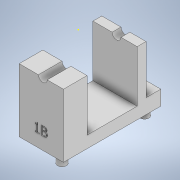
# Autodesk Inventor part: Support_1B
Saved by Autodesk Inventor 2021 (Build 250183000, 183)
## iProperties
Created: 2021-04-14
Part Number: Support_1B
Material: Generic
Document SubType Name: Modeling
Designer: Jawal
Density: 1 g/cm^3
Appearance: Default
Author: Jawal
Autodesk Inventor part; units mm, degrees
note: some values were not read from the file. Chosen so that the rebuilt part matches the saved one: direction of "Emboss1".
ref_plane "YZ Plane" through (0, 0, 0) normal (1, 0, 0) x (0, 1, 0)
ref_plane "XZ Plane" through (0, 0, 0) normal (0, 1, 0) x (-1, 0, 0)
ref_plane "XY Plane" through (0, 0, 0) normal (0, 0, 1) x (1, 0, 0)
sketch "Sketch1" plane through (0, 0, 0) normal (1, 0, 0) x (0, 1, 0)
  line L0 (12.0091, 20) -> (-9.4679, 20)
  line L1 (-9.4679, 20) -> (-9.4679, -13)
  line L2 (-9.4679, -13) -> (12.0091, -13)
  line L3 (12.0091, -13) -> (12.0091, 20)
  point P0 (0, 0)
  dimension "d0" = 33
  dimension "d1" = 21.477
  dimension "d14" = 20
  constraints: 8 end point, 2 parallel, 1 horizontal, 1 perpendicular
  measures "d0" distance of L0.end L1.end
  measures "d1" distance of L1.end L2.end
  measures "d14" distance from line of L0 point (0, 0)
extrude "Extrusion1" add sketch "Sketch1" along normal blind 15
sketch "Sketch2" plane through (0, -9.4679, -13) normal (0, -1, 0) x (1, 0, 0)
  circle A0 centre (12, 30.5) radius 1.5
  line L0 (0, 33) -> (15, 33) projected
  circle A1 centre (12, 2.5) radius 1.5
  line L1 (15, 33) -> (15, 0) projected
  point P0 (0, 13)
  dimension "d4" = 3
  dimension "d5" = 2.5
  dimension "d6" = 3
  dimension "d7" = 28
  dimension "d8" = 3
  dimension "d9" = 3
  constraints: 2 centre point
  measures "d4" diameter of A0
  measures "d5" distance from line of L0 A0.centre
  measures "d6" diameter of A1
  measures "d7" distance of A0.centre A1.centre
  measures "d8" distance from line of A1.centre L1
  measures "d9" distance from line of L1 A0.centre
extrude "Extrusion2" add sketch "Sketch2" along normal blind 3
sketch "Sketch3" plane through (15, 0, 0) normal (1, 0, 0) x (0, 0, -1)
  line L0 (13, 12.0091) -> (-20, 12.0091) projected
  line L1 (-12, 12.0091) -> (5, 12.0091)
  line L2 (5, 12.0091) -> (5, -5.48)
  line L3 (5, -5.48) -> (-12, -5.48)
  line L4 (-12, -5.48) -> (-12, 12.0091)
  line L5 (-20, 12.0091) -> (-20, -9.4679) projected
  line L6 (13, -9.4679) -> (13, 12.0091) projected
  point P0 (0, 0)
  point P1 (5, 12.0091)
  dimension "d12" = 8
  dimension "d13" = 8
  constraints: 8 end point, 2 parallel, 1 horizontal, 1 perpendicular, 1 point on line
  measures "d12" distance between parallel lines of L5 L4
  measures "d13" distance between parallel lines of L6 L2
extrude "Extrusion3" cut sketch "Sketch3" against normal through all
sketch "Sketch4" plane through (0, -9.4679, -13) normal (0, 0, -1) x (-1, 0, 0)
  line L0 (0, 21.477) -> (-15, 21.477) projected
  arc A0 (-9.517, 21.477) -> (-6.517, 21.477) centre (-8.017, 21.477) ccw
  line L1 (-15, 0) -> (-15, 21.477) projected
  point P0 (0, 9.4679)
  dimension "d17" = 3
  dimension "d18" = 6.983
  constraints: 3 point on line, 2 point on circle, 1 centre point
  measures "d17" diameter of A0
  measures "d18" distance from line of L1 A0.centre
extrude "Extrusion4" cut sketch "Sketch4" against normal through all
sketch "Sketch5" plane through (0, 12.0091, -5) normal (0, 1, 0) x (1, 0, 0)
  point P0 (0, -5)
sketch "Sketch6" plane through (0, -9.4679, -13) normal (0, 0, -1) x (-1, 0, 0)
  line L0 (-9.517, 21.477) -> (-15, 21.477) projected
  line L1 (-15, 21.477) -> (0, 21.477)
  line L2 (0, 21.477) -> (0, 5)
  line L3 (0, 5) -> (-15, 5)
  line L4 (-15, 5) -> (-15, 21.477)
  line L5 (0, 0) -> (-15, 0) projected
  point P0 (0, 9.4679)
  dimension "d21" = 5
  constraints: 8 end point, 2 parallel, 1 horizontal, 1 perpendicular
  measures "d21" distance between parallel lines of L5 L3
extrude "Extrusion5" cut sketch "Sketch6" against normal blind 5
sketch "Sketch7" plane through (0, -9.4679, 20) normal (0, 0, 1) x (1, 0, 0)
  line L0 (4.94, 7.2836) -> (14.2818, 7.2836) construction
  line L1 (14.2818, 7.2836) -> (14.2818, 1.8074) construction
  line L2 (14.2818, 1.8074) -> (4.94, 1.8074) construction
  line L3 (4.94, 1.8074) -> (4.94, 7.2836) construction
  line L4 (6.8889, 4.2257) -> (5.4019, 4.2257)
  line L5 (5.4019, 4.2257) -> (5.4019, 4.5369)
  line L6 (5.4019, 4.5369) -> (5.9552, 4.5369)
  line L7 (5.9552, 4.5369) -> (5.9552, 6.5796)
  line L8 (5.9552, 6.5796) -> (5.4019, 6.5796)
  line L9 (5.4019, 6.5796) -> (5.4019, 6.8587)
  spline S0 degree 2 poles (5.4019, 6.8587) (5.7156, 6.8587) (6.012, 7.0366) (6.0318, 7.2836) knots 0 0 0 1 2 2 2
  line L10 (6.0318, 7.2836) -> (6.3479, 7.2836)
  line L11 (6.3479, 7.2836) -> (6.3479, 4.5369)
  line L12 (6.3479, 4.5369) -> (6.8889, 4.5369)
  line L13 (6.8889, 4.5369) -> (6.8889, 4.2257)
  spline S1 degree 2 poles (9.6034, 5.1618) (9.6034, 4.9346) (9.4305, 4.5863) (9.2873, 4.4727) knots 0 0 0 1 2 2 2
  spline S2 degree 2 poles (9.2873, 4.4727) (9.1144, 4.3393) (8.7216, 4.2257) (8.4104, 4.2257) knots 0 0 0 1 2 2 2
  line L14 (8.4104, 4.2257) -> (7.536, 4.2257)
  line L15 (7.536, 4.2257) -> (7.536, 7.2737)
  line L16 (7.536, 7.2737) -> (8.3437, 7.2737)
  spline S3 degree 2 poles (8.3437, 7.2737) (8.6698, 7.2737) (8.9958, 7.2317) (9.144, 7.1502) knots 0 0 0 1 2 2 2
  spline S4 degree 2 poles (9.144, 7.1502) (9.3095, 7.0638) (9.4602, 6.7797) (9.4602, 6.587) knots 0 0 0 1 2 2 2
  spline S5 degree 2 poles (9.4602, 6.587) (9.4602, 6.3722) (9.2329, 6.0313) (9.0328, 5.935) knots 0 0 0 1 2 2 2
  line L17 (9.0328, 5.935) -> (9.0328, 5.9201)
  spline S6 degree 2 poles (9.0328, 5.9201) (9.3046, 5.846) (9.6034, 5.4533) (9.6034, 5.1618) knots 0 0 0 1 2 2 2
  spline S7 degree 2 poles (9.181, 5.1446) (9.181, 5.3175) (9.0822, 5.5398) (8.934, 5.6188) knots 0 0 0 1 2 2 2
  spline S8 degree 2 poles (8.934, 5.6188) (8.8377, 5.6682) (8.6105, 5.6978) (8.4005, 5.6978) knots 0 0 0 1 2 2 2
  line L18 (8.4005, 5.6978) -> (7.9411, 5.6978)
  line L19 (7.9411, 5.6978) -> (7.9411, 4.5715)
  line L20 (7.9411, 4.5715) -> (8.2696, 4.5715)
  spline S9 degree 2 poles (8.2696, 4.5715) (8.5364, 4.5715) (8.8427, 4.6209) (8.9612, 4.7) knots 0 0 0 1 2 2 2
  spline S10 degree 2 poles (8.9612, 4.7) (9.0748, 4.7815) (9.181, 4.984) (9.181, 5.1446) knots 0 0 0 1 2 2 2
  spline S11 degree 2 poles (9.0378, 6.5302) (9.0378, 6.6389) (8.9637, 6.8019) (8.8822, 6.8489) knots 0 0 0 1 2 2 2
  spline S12 degree 2 poles (8.8822, 6.8489) (8.7834, 6.9032) (8.5438, 6.9279) (8.3289, 6.9279) knots 0 0 0 1 2 2 2
  line L21 (8.3289, 6.9279) -> (7.9411, 6.9279)
  line L22 (7.9411, 6.9279) -> (7.9411, 6.0362)
  line L23 (7.9411, 6.0362) -> (8.4005, 6.0362)
  spline S13 degree 2 poles (8.4005, 6.0362) (8.5907, 6.0362) (8.771, 6.0758) (8.8674, 6.1375) knots 0 0 0 1 2 2 2
  spline S14 degree 2 poles (8.8674, 6.1375) (8.9612, 6.1968) (9.0378, 6.387) (9.0378, 6.5302) knots 0 0 0 1 2 2 2
  point P0 (0, 9.4679)
  constraints: 2 other
emboss "Emboss1" sketch "Sketch7" operation cut depth 1 direction (0, 0, -1)
equation "\"d9\" = d8"
body "Solid1"
